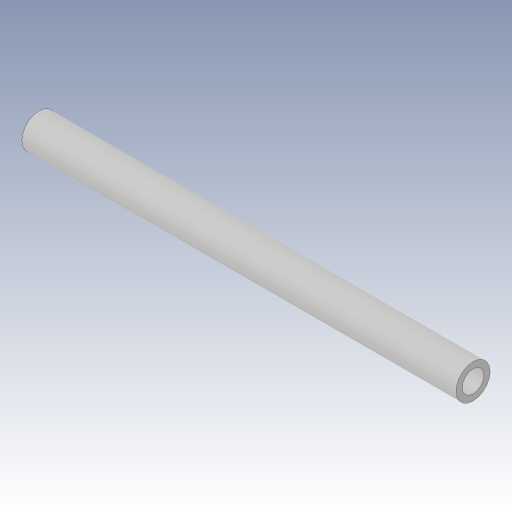
# Autodesk Inventor part: BT011_huenin20_24
Saved by Autodesk Inventor 2023.3 (Build 273359000, 359)
## iProperties
Company: HTBLA Kaindorf
RuleStatus: InUse
Created: 2024-09-13
Part Number: BT011_huenin20_24
Project: Fiberprinter-Hotend
Material: Generisch
Description: Alutube_3x0.6
Document SubType Name: Modeling
Designer: huenin20
Density: 1 g/cm^3
Appearance: Vorgabe
Mass: 0.00791681 g
Surface Area: 0.802991 cm^2
Volume: 0.00791681 cm^3
AfterDocNew0: iProperties-Editor_aufrufen
Author: nicob
Keywords: 2024
Autodesk Inventor part; units mm, degrees
ref_plane "YZ Plane" through (0, 0, 0) normal (1, 0, 0) x (0, 1, 0)
ref_plane "XZ Plane" through (0, 0, 0) normal (0, 1, 0) x (-1, 0, 0)
ref_plane "XY Plane" through (0, 0, 0) normal (0, 0, 1) x (1, 0, 0)
sketch "Skizze3" plane through (0, 0, 0) normal (0, 1, 0) x (-1, 0, 0)
  circle A0 centre (0, 0) radius 0.35
  circle A1 centre (0, 0) radius 0.55
  dimension "d4" = 0.7
  dimension "d5" = 1.1
  constraints: 2 centre point, 2 coincident
  measures "d4" diameter of A0
  measures "d5" diameter of A1
extrude "Extrusion3" add sketch "Skizze3" along normal blind 14
